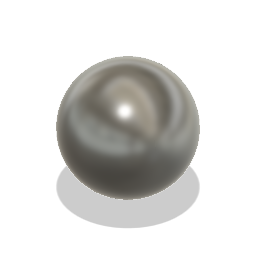
外枠 v1 (Autodesk Fusion 360 design; units mm, degrees)
Autodesk Fusion 360 part; units mm, degrees
sphere "球プリミティブ1" add diameter 100 placed x (0, 0, -1) y (0, 1, 0) z (1, 0, 0) at (0, 0, 0)
